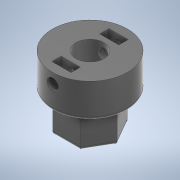
# Autodesk Inventor part: EndNut
Saved by Autodesk Inventor 2020.2 (Build 242310000, 310)
## iProperties
Created: 2021-06-25
Part Number: EndNut
Material: Generic
Document SubType Name: Modeling
Designer: JK
Density: 1 g/cm^3
Appearance: Smooth - Black
Author: JK
Autodesk Inventor part; units mm, degrees
ref_plane "YZ Plane" through (0, 0, 0) normal (1, 0, 0) x (0, 1, 0)
ref_plane "XZ Plane" through (0, 0, 0) normal (0, 1, 0) x (-1, 0, 0)
ref_plane "XY Plane" through (0, 0, 0) normal (0, 0, 1) x (1, 0, 0)
sketch "Sketch1" plane through (0, 0, 0) normal (0, 1, 0) x (-1, 0, 0)
  line L0 (12.7017, 0) -> (6.3509, -11)
  line L1 (6.3509, -11) -> (-6.3509, -11)
  line L2 (-6.3509, -11) -> (-12.7017, 0)
  line L3 (-12.7017, 0) -> (-6.3509, 11)
  line L4 (-6.3509, 11) -> (6.3509, 11)
  line L5 (6.3509, 11) -> (12.7017, 0)
  circle A0 centre (0, 0) radius 11
  circle A1 centre (0, 0) radius 4.1
  dimension "d0" = 22
  dimension "d1" = 8.2
  constraints: 12 end point, 3 coincident, 2 centre point, 1 tangent, 13 other
  measures "d0" diameter of A0
  measures "d1" diameter of A1
extrude "Extrusion1" add sketch "Sketch1" along normal blind 8
sketch "Sketch2" plane through (0, 8, 0) normal (0, 1, 0) x (1, 0, 0)
  line L0 (-2.8, -8.35) -> (2.8, -8.35)
  line L1 (2.8, -8.35) -> (2.8, -5.65)
  line L2 (2.8, -5.65) -> (-2.8, -5.65)
  line L3 (-2.8, -5.65) -> (-2.8, -8.35)
  line L4 (-2.8, -8.35) -> (2.8, -5.65) construction
  line L5 (2.8, -8.35) -> (-2.8, -5.65) construction
  point P0 (0, 0)
  point P1 (0, -7)
  point P2 (0, -7)
  dimension "d4" = 2.7
  dimension "d5" = 5.6
  dimension "d8" = 7
  constraints: 12 end point, 3 midpoint, 2 parallel, 1 horizontal, 1 perpendicular, 1 vertical alignment
  measures "d4" distance of L2.end L0.start
  measures "d5" distance of L1.end L2.end
  measures "d8" distance of point (0, -7) point (0, 0)
extrude "Extrusion2" cut sketch "Sketch2" against normal blind 6.5
mirror "Mirror1" about plane through (0, 0, 0) normal (0, 0, 1) of "Extrusion2"
sketch "Sketch3" plane through (6.3509, 0, -11) normal (0, 0, -1) x (-1, 0, 0)
  circle A0 centre (6.3509, 5) radius 1.6
  line L0 (0, 0) -> (12.7017, 0) projected
  point P0 (6.3509, 0)
  point P1 (6.3509, 0)
  dimension "d9" = 3.2
  dimension "d10" = 5
  constraints: 1 centre point, 1 midpoint, 1 vertical alignment
  measures "d9" diameter of A0
  measures "d10" distance of point (6.351, 0) A0.centre
extrude "Extrusion3" cut sketch "Sketch3" against normal through all
sketch "Sketch5" plane through (0, 0, 0) normal (0, -1, 0) x (1, 0, 0)
  circle A0 centre (0, 0) radius 11
  line L0 (6.3509, -11) -> (-6.3509, -11) projected
  circle A1 centre (0, 0) radius 14.2349
  constraints: 2 centre point, 2 coincident, 1 tangent
extrude "Extrusion5" cut sketch "Sketch5" against normal through all
sketch "Sketch6" plane through (0, 0, 0) normal (0, -1, 0) x (1, 0, 0)
  circle A0 centre (0, 0) radius 11 projected
  circle A1 centre (0, 0) radius 4.1 projected
extrude "Extrusion6" add sketch "Sketch6" along normal blind 2
sketch "Sketch7" plane through (0, -2, 0) normal (0, -1, 0) x (1, 0, 0)
  line L0 (-7.9674, 0) -> (-3.9837, 6.9)
  line L1 (-3.9837, 6.9) -> (3.9837, 6.9)
  line L2 (3.9837, 6.9) -> (7.9674, 0)
  line L3 (7.9674, 0) -> (3.9837, -6.9)
  line L4 (3.9837, -6.9) -> (-3.9837, -6.9)
  line L5 (-3.9837, -6.9) -> (-7.9674, 0)
  circle A0 centre (0, 0) radius 6.9
  circle A1 centre (0, 0) radius 4.1 projected
  dimension "d19" = 13.8
  constraints: 12 end point, 2 coincident, 1 centre point, 1 tangent, 13 other
  measures "d19" diameter of A0
extrude "Extrusion7" add sketch "Sketch7" along normal blind 10
sketch "Sketch8" plane through (0, -12, 0) normal (0, -1, 0) x (1, 0, 0)
  circle A0 centre (0, 0) radius 4.1
  constraints: 1 centre point, 1 coincident
extrude "Extrusion8" add sketch "Sketch8" against normal blind 2
fillet "Fillet1" radius 1 6 edges at (0, -12, -6.9) (-5.9756, -12, -3.45) (-5.9756, -12, 3.45) (0, -12, 6.9) (5.9756, -12, 3.45) (5.9756, -12, -3.45)
fillet "Fillet2" radius 1 1 edges at (-11, -2, 0)
sketch "Sketch4" plane through (0, 0, 0) normal (0, -1, 0) x (1, 0, 0)
  line L0 (-2.8, -5.25) -> (2.8, -5.25) projected
  line L1 (2.8, -5.25) -> (2.8, -7.95) projected
  line L2 (2.8, -7.95) -> (-2.8, -7.95) projected
  line L3 (-2.8, -7.95) -> (-2.8, -5.25) projected
  line L4 (2.8, 5.25) -> (-2.8, 5.25) projected
  line L5 (-2.8, 5.25) -> (-2.8, 7.95) projected
  line L6 (-2.8, 7.95) -> (2.8, 7.95) projected
  line L7 (2.8, 7.95) -> (2.8, 5.25) projected
  line L8 (5.4848, -9.5) -> (-5.4848, -9.5) projected
  line L9 (10.9697, 0) -> (5.4848, -9.5) projected
  line L10 (5.4848, 9.5) -> (10.9697, 0) projected
  line L11 (-5.4848, 9.5) -> (5.4848, 9.5) projected
  line L12 (-10.9697, 0) -> (-5.4848, 9.5) projected
  line L13 (-5.4848, -9.5) -> (-10.9697, 0) projected
  circle A0 centre (0, 0) radius 4.1 projected
body "Solid1"
